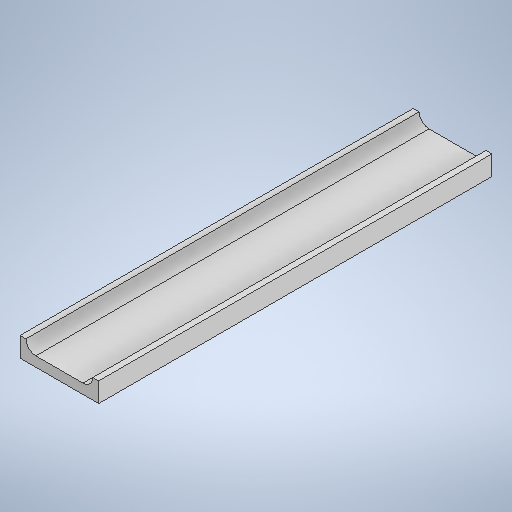
# Autodesk Inventor part: Part3
Saved by Autodesk Inventor 2025.4 (Build 294407000, 407)
## iProperties
Created: 2026-03-03
Part Number: Part3
Material: Generic
Document SubType Name: Modeling
Designer: Amir
Density: 1 g/cm^3
Appearance: Default
Author: Amir
Autodesk Inventor part; units mm, degrees
ref_plane "YZ Plane" through (0, 0, 0) normal (1, 0, 0) x (0, 1, 0)
ref_plane "XZ Plane" through (0, 0, 0) normal (0, 1, 0) x (-1, 0, 0)
ref_plane "XY Plane" through (0, 0, 0) normal (0, 0, 1) x (1, 0, 0)
sketch "Sketch1" plane through (0, 0, 0) normal (0, 0, 1) x (1, 0, 0)
  line L0 (-20, -7.5) -> (20, -7.5)
  line L1 (20, -7.5) -> (20, 2.5)
  line L2 (-20, 2.5) -> (-20, -7.5)
  line L3 (-17, -2.5) -> (-17, 2.5)
  line L4 (17, 2.5) -> (17, -2.5)
  line L5 (-21.1547, 2.5) -> (25.819, 2.5)
  line L6 (-17, -2.5) -> (17, -2.5)
  point P0 (0, 0)
  point P1 (0, -7.5)
  dimension "d2" = 3
  dimension "d7" = 40
  dimension "d8" = 3
  dimension "d9" = 10
  dimension "d10" = 5
  dimension "d17" = 34
  dimension "d18" = 5
  constraints: 14 end point, 4 point on line, 3 horizontal, 2 parallel, 1 midpoint, 1 perpendicular
  measures "d2" distance between parallel lines of L2 L3
  measures "d7" distance of L0.start L0.end
  measures "d8" distance between parallel lines of L1 L4
  measures "d9" distance of L2.start L0.start
  measures "d10" distance of L3.start L3.end
  measures "d17" distance between parallel lines of L4 L3
  measures "d18" distance between parallel lines of L0 L6
extrude "Extrusion3" add sketch "Sketch1" along normal blind 200 contours L2 L5 L3 L6 L4 L1 L0
fillet "Fillet3" radius 5 1 edges at (-17, -2.5, 100)
fillet "Fillet4" radius 5 1 edges at (17, -2.5, 100)
body "Solid3"
